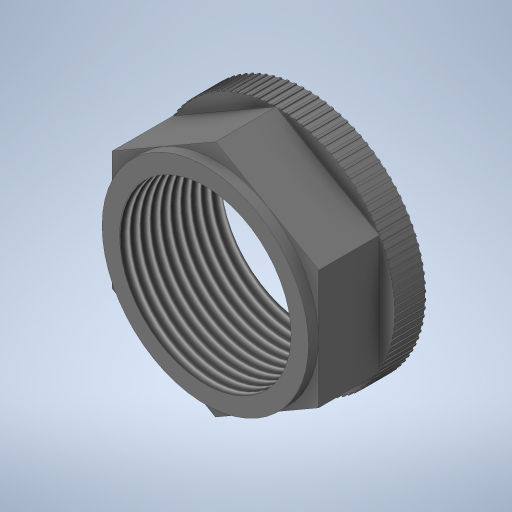
# Autodesk Inventor part: 2309HCMUTE-CDT23-CB_CLAMP-NUT
Saved by Autodesk Inventor 2023 (Build 270158000, 158)
## iProperties
Created: 2023-10-11
Part Number: 2309HCMUTE-CDT23-CB_CLAMP-NUT
Material: PPS Plastic
Document SubType Name: Modeling
Designer: havie
Density: 1.637 g/cm^3
Appearance: Gray
Author: havie
Autodesk Inventor part; units mm, degrees
ref_plane "YZ Plane" through (0, 0, 0) normal (1, 0, 0) x (0, 1, 0)
ref_plane "XZ Plane" through (0, 0, 0) normal (0, 1, 0) x (-1, 0, 0)
ref_plane "XY Plane" through (0, 0, 0) normal (0, 0, 1) x (1, 0, 0)
sketch "Sketch1" plane through (0, 0, 0) normal (0, 1, 0) x (-1, 0, 0)
  circle A0 centre (0, 0) radius 11.75
  dimension "d0" = 23.5
  constraints: 1 centre point, 1 coincident
  measures "d0" diameter of A0
extrude "Extrusion1" add sketch "Sketch1" along normal mid plane 3
sketch "Sketch2" plane through (0, -1.5, 0) normal (0, -1, 0) x (1, 0, 0)
  line L0 (11.85, 0.25) -> (11.65, 0.25)
  line L1 (11.65, 0.25) -> (11.65, -0.25)
  line L2 (11.65, -0.25) -> (11.85, -0.25)
  line L3 (11.85, -0.25) -> (11.85, 0.25)
  line L4 (-16.47, 0) -> (16.57, 0) projected
  circle A0 centre (0, 0) radius 11.75 projected
  point P0 (11.7473, 0.25)
  point P1 (11.7473, -0.25)
  dimension "d3" = 0.5
  dimension "d11" = 0.2
  dimension "d12" = 0.1
  constraints: 8 end point, 2 parallel, 1 horizontal, 1 perpendicular, 1 other
  measures "d3" distance between parallel lines of L2 L0
  measures "d11" distance between parallel lines of L3 L1
  measures "d12" distance edge to line of A0 L1
extrude "Extrusion2" cut sketch "Sketch2" against normal through all contours A0 L4 L1 L0 | A0 L2 L1 L4 picked at (11.6829, 0.1389) picked at (11.6829, -0.1389)
pattern_circular "Circular Pattern1" count 100 over 360 about axis through (0, -10, 0) along (0, 1, 0) of "Extrusion2"
sketch "Sketch3" plane through (0, -1.5, 0) normal (0, -1, 0) x (1, 0, 0)
  line L0 (0, -11.75) -> (-10.1758, -5.875)
  line L1 (-10.1758, -5.875) -> (-10.1758, 5.875)
  line L2 (-10.1758, 5.875) -> (0, 11.75)
  line L3 (0, 11.75) -> (10.1758, 5.875)
  line L4 (10.1758, 5.875) -> (10.1758, -5.875)
  line L5 (10.1758, -5.875) -> (0, -11.75)
  arc A0 (0.4881, 11.7399) -> (0.25, 11.7473) centre (0, 0) ccw construction
  circle A1 centre (0, 0) radius 11.75 construction
  constraints: 12 end point, 2 coincident, 2 point on circle, 1 centre point, 1 vertical alignment, 13 other
extrude "Extrusion3" add sketch "Sketch3" along normal blind 7
sketch "Sketch4" plane through (0, -8.5, 0) normal (0, -1, 0) x (1, 0, 0)
  point P0 (0, 0)
  point P1 (0, 0)
  constraints: 1 coincident
hole "Hole1" at (0, -8.5, 0) direction (0, 1, 0) diameter 16.9175 end through all thread size "M18x1" class "6H" standard "ISO Metric profile"
sketch "Sketch5" plane through (0, -8.5, 0) normal (0, -1, 0) x (1, 0, 0)
  circle A0 centre (0, 0) radius 10.1758
  line L0 (-10.1758, -5.875) -> (0, -11.75) projected
  line L1 (0, 11.75) -> (-10.1758, 5.875) projected
  line L2 (-10.1758, 5.875) -> (-10.1758, -5.875) projected
  line L3 (10.1758, 5.875) -> (0, 11.75) projected
  line L4 (10.1758, -5.875) -> (10.1758, 5.875) projected
  line L5 (0, -11.75) -> (10.1758, -5.875) projected
  point P0 (5.0879, -8.8125)
  point P1 (-5.0879, -8.8125)
  point P2 (10.1758, 0)
  point P3 (5.0879, 8.8125)
  point P4 (-10.1758, 0)
  point P5 (-5.0879, 8.8125)
  constraints: 1 centre point, 1 coincident, 1 tangent
extrude "Extrusion4" cut sketch "Sketch5" against normal blind 1 contours L4 L5 A0 | A0 L3 L4 | A0 L1 L3 | L5 L0 A0 | A0 L2 L1 | L0 L2 A0
body "Solid1"
